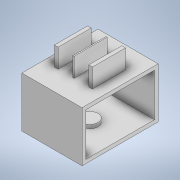
# Autodesk Inventor part: Koszyk
Saved by Autodesk Inventor 2020 (Build 240168000, 168)
## iProperties
Created: 2020-03-14
Part Number: Koszyk
Material: Generic
Document SubType Name: Modeling
Designer: atmat
Density: 1 g/cm^3
Appearance: Default
Author: atmat
Autodesk Inventor part; units mm, degrees
ref_plane "YZ Plane" through (0, 0, 0) normal (1, 0, 0) x (0, 1, 0)
ref_plane "XZ Plane" through (0, 0, 0) normal (0, 1, 0) x (-1, 0, 0)
ref_plane "XY Plane" through (0, 0, 0) normal (0, 0, 1) x (1, 0, 0)
sketch "Sketch1" plane through (0, 0, 0) normal (0, 1, 0) x (-1, 0, 0)
  line L0 (-0.5, 13.5) -> (-12.5, 13.5)
  line L1 (-12.5, 13.5) -> (-12.5, -13.5)
  line L2 (-12.5, -13.5) -> (-0.5, -13.5)
  line L3 (-0.5, -13.5) -> (-0.5, 13.5)
  line L4 (12.5, 13.5) -> (0.5, 13.5)
  line L5 (0.5, 13.5) -> (0.5, -13.5)
  line L6 (0.5, -13.5) -> (12.5, -13.5)
  line L7 (12.5, -13.5) -> (12.5, 13.5)
  line L8 (15.5, 13.5) -> (-15.5, 13.5)
  line L9 (-15.5, 13.5) -> (-15.5, -13.5)
  line L10 (-15.5, -13.5) -> (15.5, -13.5)
  line L11 (15.5, -13.5) -> (15.5, 13.5)
  point P0 (0, 0)
  point P1 (-0.5, -13.5)
  point P2 (0.5, -13.5)
  point P3 (0.5, 13.5)
  dimension "d0" = 12
  dimension "d1" = 12
  dimension "d2" = 1
  dimension "d3" = 27
  dimension "d4" = 27
  dimension "d5" = 0
  dimension "d6" = 0.5
  dimension "d7" = 13.5
  dimension "d8" = 3
  dimension "d9" = 3
  dimension "d10" = 0
  dimension "d11" = 0
  constraints: 24 end point, 6 parallel, 3 horizontal, 3 perpendicular
  measures "d0" distance of L4.start L4.end
  measures "d1" distance of L0.start L0.end
  measures "d2" distance between parallel lines of L5 L3
  measures "d3" distance of L6.end L4.start
  measures "d4" distance of L0.end L1.end
  measures "d5" distance between parallel lines of L4 L0
  measures "d6" distance from line of point (0, 0) L3
  measures "d7" distance from line of point (0, 0) L0
  measures "d8" distance between parallel lines of L7 L11
  measures "d9" distance between parallel lines of L1 L9
  measures "d10" distance between parallel lines of L4 L8
  measures "d11" distance between parallel lines of L10 L6
extrude "Extrusion1" add sketch "Sketch1" along normal blind 15.5 contours L8 L5 L10 L3 | L1 L10 L9 L8 | L8 L11 L10 L7
sketch "Sketch2" plane through (0, 0, 0) normal (0, -1, 0) x (1, 0, 0)
  line L0 (24.5, 28) -> (-24.5, 28)
  line L1 (-24.5, 28) -> (-24.5, -28)
  line L2 (-24.5, -28) -> (24.5, -28)
  line L3 (24.5, -28) -> (24.5, 28)
  line L4 (15.5, 13.5) -> (15.5, -13.5) projected
  line L5 (-15.5, -13.5) -> (-15.5, 13.5) projected
  line L6 (24.5, 28) -> (-24.5, 28)
  line L7 (-24.5, 28) -> (-24.5, 31)
  line L8 (-24.5, 31) -> (24.5, 31)
  line L9 (24.5, 31) -> (24.5, 28)
  line L10 (-24.5, -28) -> (24.5, -28)
  line L11 (24.5, -28) -> (24.5, -31)
  line L12 (24.5, -31) -> (-24.5, -31)
  line L13 (-24.5, -31) -> (-24.5, -28)
  point P0 (0, 0)
  point P1 (24.5, -28)
  point P2 (-24.5, 28)
  dimension "d14" = 56
  dimension "d15" = 28
  dimension "d16" = 9
  dimension "d17" = 9
  dimension "d18" = 3
  dimension "d19" = 3
  constraints: 24 end point, 6 parallel, 3 horizontal, 3 perpendicular, 1 point on line
  measures "d14" distance of L2.end L0.start
  measures "d15" distance from line of point (0, 0) L0
  measures "d16" distance between parallel lines of L4 L3
  measures "d17" distance between parallel lines of L1 L5
  measures "d18" distance between parallel lines of L6 L8
  measures "d19" distance between parallel lines of L10 L12
extrude "Extrusion2" add sketch "Sketch2" along normal blind 3
sketch "Sketch3" plane through (0, -3, 0) normal (0, -1, 0) x (1, 0, 0)
  line L0 (24.5, 28) -> (-24.5, 28)
  line L1 (-24.5, 28) -> (-24.5, -28)
  line L2 (-24.5, -28) -> (24.5, -28)
  line L3 (24.5, -28) -> (24.5, 28)
  line L4 (24.5, 28) -> (-24.5, 28)
  line L5 (-24.5, 28) -> (-24.5, 31)
  line L6 (-24.5, 31) -> (24.5, 31)
  line L7 (24.5, 31) -> (24.5, 28)
  line L8 (-24.5, -28) -> (24.5, -28)
  line L9 (24.5, -28) -> (24.5, -31)
  line L10 (24.5, -31) -> (-24.5, -31)
  line L11 (-24.5, -31) -> (-24.5, -28)
  point P0 (0, 0)
  point P1 (24.5, -28)
  point P2 (-24.5, 28)
  point P3 (-24.5, 28)
  point P4 (24.5, -28)
  dimension "d22" = 56
  dimension "d23" = 28
  dimension "d26" = 3
  dimension "d27" = 3
  constraints: 24 end point, 6 parallel, 3 horizontal, 3 perpendicular, 1 point on line
  measures "d22" distance of L2.end L0.start
  measures "d23" distance from line of point (0, 0) L0
  measures "d26" distance between parallel lines of L4 L6
  measures "d27" distance between parallel lines of L8 L10
extrude "Extrusion3" add sketch "Sketch3" along normal blind 35 contours L0 L5 L6 L7 | L9 L10 L11 L2
sketch "Sketch4" plane through (0, -38, 0) normal (0, -1, 0) x (1, 0, 0)
  line L0 (24.5, 28) -> (-24.5, 28)
  line L1 (-24.5, 28) -> (-24.5, -28)
  line L2 (-24.5, -28) -> (24.5, -28)
  line L3 (24.5, -28) -> (24.5, 28)
  line L4 (24.5, 28) -> (-24.5, 28)
  line L5 (-24.5, 28) -> (-24.5, 31)
  line L6 (-24.5, 31) -> (24.5, 31)
  line L7 (24.5, 31) -> (24.5, 28)
  line L8 (-24.5, -28) -> (24.5, -28)
  line L9 (24.5, -28) -> (24.5, -31)
  line L10 (24.5, -31) -> (-24.5, -31)
  line L11 (-24.5, -31) -> (-24.5, -28)
  point P0 (0, 0)
  point P1 (24.5, -28)
  point P2 (-24.5, 28)
  dimension "d30" = 56
  dimension "d31" = 28
  dimension "d34" = 3
  dimension "d35" = 3
  constraints: 24 end point, 6 parallel, 3 horizontal, 3 perpendicular, 1 point on line
  measures "d30" distance of L2.end L0.start
  measures "d31" distance from line of point (0, 0) L0
  measures "d34" distance between parallel lines of L4 L6
  measures "d35" distance between parallel lines of L8 L10
extrude "Extrusion4" add sketch "Sketch4" along normal blind 3
sketch "Sketch7" plane through (0, -41, 0) normal (0, -1, 0) x (1, 0, 0)
  circle A0 centre (0, 0) radius 6.5
  dimension "d45" = 13
  constraints: 1 centre point, 1 coincident
  measures "d45" diameter of A0
extrude "Extrusion7" add sketch "Sketch7" against normal blind 6
sketch "Sketch8" plane through (0, -41, 0) normal (0, -1, 0) x (1, 0, 0)
  circle A0 centre (0, 0) radius 3.75
  circle A1 centre (0, 0) radius 5
  dimension "d48" = 7.5
  dimension "d49" = 10
  constraints: 2 centre point, 2 coincident
  measures "d48" diameter of A0
  measures "d49" diameter of A1
extrude "Extrusion8" cut sketch "Sketch8" against normal blind 5
sketch "Sketch9" plane through (0, -41, 0) normal (0, -1, 0) x (1, 0, 0)
  circle A0 centre (0, 0) radius 3.75
  circle A1 centre (0, 0) radius 5
  circle A2 centre (0, 0) radius 6.5
  dimension "d52" = 13
  dimension "d53" = 10
  dimension "d54" = 7.5
  constraints: 3 centre point, 3 coincident
  measures "d52" diameter of A2
  measures "d53" diameter of A1
  measures "d54" diameter of A0
extrude "Extrusion9" add sketch "Sketch9" along normal blind 5
body "Solid1"
